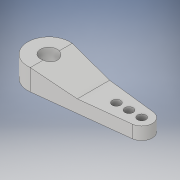
# Autodesk Inventor part: ServoArm 22mm
Saved by Autodesk Inventor 2018.2 (Build 222227000, 227)
## iProperties
Created: 2018-02-17
Part Number: ServoArm 22mm
Material: Generisch
Document SubType Name: Modeling
Designer: JochenAlt
Density: 1 g/cm^3
Appearance: Vorgabe
Author: JochenAlt
Autodesk Inventor part; units mm, degrees
note: some values were not read from the file. Chosen so that the rebuilt part matches the saved one: sketch regions of "Extrusion1".
ref_plane "YZ Plane" through (0, 0, 0) normal (1, 0, 0) x (0, 1, 0)
ref_plane "XZ Plane" through (0, 0, 0) normal (0, 1, 0) x (-1, 0, 0)
ref_plane "XY Plane" through (0, 0, 0) normal (0, 0, 1) x (1, 0, 0)
sketch "Skizze1" plane through (0, 0, 0) normal (0, 0, 1) x (1, 0, 0)
  line L0 (0, 7) -> (0, -7) construction
  line L1 (-10.9, 0) -> (30.4, 0) construction
  circle A0 centre (0, 0) radius 2
  circle A1 centre (16, 0) radius 1
  circle A2 centre (19, 0) radius 1
  circle A3 centre (22, 0) radius 1
  arc A4 (22.2841, -2.4838) -> (22.2841, 2.4838) centre (22, 0) ccw
  arc A5 (0.5682, 4.9676) -> (0.5682, -4.9676) centre (0, 0) ccw
  line L2 (0.5682, 4.9676) -> (22.2841, 2.4838)
  line L3 (0.5682, -4.9676) -> (22.2841, -2.4838)
  line L4 (0.5682, -4.9676) -> (0.5682, -1.9176)
  line L5 (0.5682, 1.9176) -> (0.5682, 4.9676)
  line L6 (0.5682, 1.9176) -> (0.5682, -1.9176)
  dimension "d1" = 19
  dimension "d2" = 22
  dimension "d3" = 5
  dimension "d4" = 2
  dimension "d5" = 4
  dimension "d6" = 10
  dimension "d16" = 16
  constraints: 10 end point, 7 point on circle, 6 centre point, 4 tangent, 3 coincident, 3 point on line, 2 equal radius, 1 collinear, 1 vertical
  measures "d1" distance of point (0, 0) A2.centre
  measures "d2" distance of A3.centre point (0, 0)
  measures "d3" diameter of A4
  measures "d4" diameter of A3
  measures "d5" diameter of A0
  measures "d6" diameter of A5
  measures "d16" distance of point (0, 0) A1.centre
extrude "Extrusion1" add sketch "Skizze1" along normal blind 3
extrude "Extrusion2" add sketch "Skizze1" along normal blind 5 contours L6 A0 | A0 L4 A5 L5 picked at (-0.8876, -0.1748)
chamfer "Fase1" distance 10 distance2 2 1 edges at (0.5682, 0, 3) measured on face at (5.3788, 0, 3)
extrude "Extrusion3" cut sketch "Skizze1" along normal blind 5 contours A0 L6 | L6 A0
